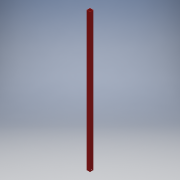
# Autodesk Inventor part: climb bar
Saved by Autodesk Inventor 2017 SP1 (Build 210196100, 196)
## iProperties
Created: 2018-03-18
Part Number: climb bar
Material: Generic
Document SubType Name: Modeling
Designer: Ben
Density: 1 g/cm^3
Appearance: Light Red
Mass: 145.847 g
Surface Area: 1841.1 cm^2
Volume: 145.847 cm^3
Author: Ben
Autodesk Inventor part; units mm, degrees
ref_plane "YZ Plane" through (0, 0, 0) normal (1, 0, 0) x (0, 1, 0)
ref_plane "XZ Plane" through (0, 0, 0) normal (0, 1, 0) x (-1, 0, 0)
ref_plane "XY Plane" through (0, 0, 0) normal (0, 0, 1) x (1, 0, 0)
sketch "Sketch1" plane through (0, 0, 0) normal (0, 1, 0) x (-1, 0, 0)
  line L0 (-12.7, 12.7) -> (12.7, 12.7)
  line L1 (12.7, 12.7) -> (12.7, -12.7)
  line L2 (12.7, -12.7) -> (-12.7, -12.7)
  line L3 (-12.7, -12.7) -> (-12.7, 12.7)
  line L4 (-12.7, 12.7) -> (12.7, -12.7) construction
  line L5 (12.7, 12.7) -> (-12.7, -12.7) construction
  line L6 (11.1125, -11.1125) -> (11.1125, 11.1125)
  line L7 (11.1125, 11.1125) -> (-11.1125, 11.1125)
  line L8 (-11.1125, 11.1125) -> (-11.1125, -11.1125)
  line L9 (-11.1125, -11.1125) -> (11.1125, -11.1125)
  point P0 (0, 0)
  dimension "d0" = 25.4
  dimension "d1" = 1.5875
  constraints: 20 end point, 4 parallel, 3 perpendicular, 2 midpoint, 1 horizontal, 3 other
  measures "d0" distance of L1.end L2.end
  measures "d1" distance between parallel lines of L1 L6
extrude "Extrusion1" add sketch "Sketch1" along normal mid plane 1016
sketch "Sketch2" plane through (12.7, -508, -12.7) normal (1, 0, 0) x (0, 0, -1)
  circle A0 centre (-12.7, 9.525) radius 3.175
  line L0 (-12.7, 9.525) -> (-12.7, 0) construction
  line L1 (-23.8125, 0) -> (-1.5875, 0) construction
  point P0 (-12.7, 508)
  dimension "d4" = 6.35
  dimension "d5" = 9.525
  constraints: 2 end point, 1 centre point, 1 midpoint, 1 vertical
  measures "d4" diameter of A0
  measures "d5" distance of L0.start L0.end
extrude "Extrusion2" cut sketch "Sketch2" against normal through all
body "Solid1"
